# Autodesk Inventor part: PQ60 EPS FV4.brd_Outline
Saved by Autodesk Inventor 2015 SP1 (Build 190203100, 203)
## iProperties
Created: 2015-10-19
Part Number: PQ60 EPS FV4.brd_Outline
Material: Generic
Document SubType Name: Modeling
Designer: Kartikye
Density: 1 g/cm^3
Appearance: Board Outline
Author: Kartikye
Autodesk Inventor part; units mm, degrees
ref_plane "YZ Plane" through (0, 0, 0) normal (1, 0, 0) x (0, 1, 0)
ref_plane "XZ Plane" through (0, 0, 0) normal (0, 1, 0) x (-1, 0, 0)
ref_plane "XY Plane" through (0, 0, 0) normal (0, 0, 1) x (1, 0, 0)
sketch "Sketch1" plane through (0, 0, 0) normal (0, 0, 1) x (1, 0, 0)
  line L0 (42, 3) -> (42, 39)
  line L1 (42, 39) -> (41.8978, 39.7765)
  line L2 (41.8978, 39.7765) -> (41.5981, 40.5)
  line L3 (41.5981, 40.5) -> (41.1213, 41.1213)
  line L4 (41.1213, 41.1213) -> (40.5, 41.5981)
  line L5 (40.5, 41.5981) -> (39.7765, 41.8978)
  line L6 (39.7765, 41.8978) -> (39, 42)
  line L7 (39, 42) -> (3, 42)
  line L8 (3, 42) -> (2.2235, 41.8978)
  line L9 (2.2235, 41.8978) -> (1.5, 41.5981)
  line L10 (1.5, 41.5981) -> (0.8787, 41.1213)
  line L11 (0.8787, 41.1213) -> (0.4019, 40.5)
  line L12 (0.4019, 40.5) -> (0.1022, 39.7765)
  line L13 (0.1022, 39.7765) -> (0, 39)
  line L14 (0, 39) -> (0, 3)
  line L15 (0, 3) -> (0.1022, 2.2235)
  line L16 (0.1022, 2.2235) -> (0.4019, 1.5)
  line L17 (0.4019, 1.5) -> (0.8787, 0.8787)
  line L18 (0.8787, 0.8787) -> (1.5, 0.4019)
  line L19 (1.5, 0.4019) -> (2.2235, 0.1022)
  line L20 (2.2235, 0.1022) -> (3, 0)
  line L21 (3, 0) -> (39, 0)
  line L22 (39, 0) -> (39.7765, 0.1022)
  line L23 (39.7765, 0.1022) -> (40.5, 0.4019)
  line L24 (40.5, 0.4019) -> (41.1213, 0.8787)
  line L25 (41.1213, 0.8787) -> (41.5981, 1.5)
  line L26 (41.5981, 1.5) -> (41.8978, 2.2235)
  line L27 (41.8978, 2.2235) -> (42, 3)
  circle A0 centre (32.1, 8.8) radius 0.55
  circle A1 centre (9.9, 8.8) radius 0.35
  circle A2 centre (32.1, 8.5) radius 0.55
  circle A3 centre (9.9, 8.5) radius 0.35
  circle A4 centre (14.1, 12.1) radius 0.15
  circle A5 centre (16, 13.35) radius 0.15
  circle A6 centre (29.7, 2.6) radius 0.15
  circle A7 centre (35.3, 30.85) radius 0.15
  circle A8 centre (11.6, 12.1) radius 0.15
  circle A9 centre (11.6, 13.7) radius 0.15
  circle A10 centre (40.65, 7.95) radius 0.15
  circle A11 centre (14.85, 15.6) radius 0.15
  circle A12 centre (12.025, 26.75) radius 0.15
  circle A13 centre (12.025, 32.45) radius 0.15
  circle A14 centre (23.75, 32.425) radius 0.15
  circle A15 centre (30.6, 9.2) radius 0.15
  circle A16 centre (27.75, 11.25) radius 0.15
  circle A17 centre (24.9, 11.3) radius 0.15
  circle A18 centre (37.05, 26.85) radius 0.15
  circle A19 centre (24.9, 1.8) radius 0.15
  circle A20 centre (13.5, 12.9) radius 0.15
  circle A21 centre (17.1, 11.975) radius 0.15
  circle A22 centre (20.2, 11.975) radius 0.15
  circle A23 centre (23.3, 11.975) radius 0.15
  circle A24 centre (10.9, 12.9) radius 0.15
  circle A25 centre (22.5, 11.25) radius 0.15
  circle A26 centre (19.5, 11.3) radius 0.15
  circle A27 centre (17.7, 11.25) radius 0.15
  circle A28 centre (19.15, 25.175) radius 0.15
  circle A29 centre (3, 39) radius 1
  circle A30 centre (3, 3) radius 1
  circle A31 centre (39, 3) radius 1
  circle A32 centre (31.1, 7.05) radius 0.15
  circle A33 centre (7, 7.05) radius 0.15
  circle A34 centre (5.6, 7.05) radius 0.15
  circle A35 centre (13.5, 11.3) radius 0.15
  circle A36 centre (10.375, 36.875) radius 0.15
  circle A37 centre (20.85, 36.95) radius 0.15
  circle A38 centre (24.9, 36.275) radius 0.15
  circle A39 centre (30.55, 36.7) radius 0.15
  circle A40 centre (6, 18.6) radius 0.15
  circle A41 centre (30.95, 24.55) radius 0.15
  circle A42 centre (34.8, 23.4) radius 0.15
  circle A43 centre (10.9, 23.3) radius 0.15
  circle A44 centre (8.75, 23.4) radius 0.15
  circle A45 centre (14.2, 24.6) radius 0.15
  circle A46 centre (14.1, 22.25) radius 0.15
  circle A47 centre (18, 13.35) radius 0.15
  circle A48 centre (21.1, 13.35) radius 0.15
  circle A49 centre (16, 16.15) radius 0.15
  circle A50 centre (13.9, 14.3) radius 0.15
  circle A51 centre (19.375, 15.975) radius 0.15
  circle A52 centre (24.25, 13.4) radius 0.15
  circle A53 centre (27.35, 13.35) radius 0.15
  circle A54 centre (30.35, 12.1) radius 0.15
  circle A55 centre (34.9, 14.1) radius 0.15
  circle A56 centre (35.25, 7.7) radius 0.15
  circle A57 centre (40.675, 13.725) radius 0.15
  circle A58 centre (34.475, 21.275) radius 0.15
  circle A59 centre (38.225, 13.95) radius 0.15
  circle A60 centre (22.325, 27.6) radius 0.15
  circle A61 centre (9.8, 26.075) radius 0.15
  circle A62 centre (13.175, 27.15) radius 0.15
  circle A63 centre (27, 19.525) radius 0.15
  circle A64 centre (23.875, 15.75) radius 0.15
  circle A65 centre (29.525, 21.15) radius 0.15
  circle A66 centre (29.475, 27.45) radius 0.15
  circle A67 centre (31.675, 0.775) radius 0.15
  circle A68 centre (2.45, 8.075) radius 0.15
  circle A69 centre (39, 26.85) radius 0.15
  circle A70 centre (11.975, 35.375) radius 0.15
  circle A71 centre (6.2, 36.55) radius 0.15
  circle A72 centre (25.2, 32.45) radius 0.15
  circle A73 centre (34.5, 36.7) radius 0.15
  circle A74 centre (13.1, 30.875) radius 0.15
  circle A75 centre (6.6, 14.5) radius 0.15
  circle A76 centre (20.7, 2.7) radius 0.15
  circle A77 centre (9.05, 27.55) radius 0.15
  circle A78 centre (14.1, 19) radius 0.15
  circle A79 centre (15.3, 12.025) radius 0.15
  circle A80 centre (14.7, 11.3) radius 0.15
  circle A81 centre (14.1, 1.9) radius 0.15
  circle A82 centre (14.7, 2.7) radius 0.15
  circle A83 centre (15.3, 1.9) radius 0.15
  circle A84 centre (15.9, 2.7) radius 0.15
  circle A85 centre (16.5, 1.9) radius 0.15
  circle A86 centre (17.1, 2.7) radius 0.15
  circle A87 centre (17.7, 1.9) radius 0.15
  circle A88 centre (18.3, 2.7) radius 0.15
  circle A89 centre (18.9, 1.9) radius 0.15
  circle A90 centre (19.5, 2.7) radius 0.15
  circle A91 centre (20.1, 1.9) radius 0.15
  circle A92 centre (12.9, 1.9) radius 0.15
  circle A93 centre (12.2977, 2.7) radius 0.15
  circle A94 centre (19.8, 35.7) radius 0.15
  circle A95 centre (31.525, 35.675) radius 0.15
  circle A96 centre (9.05, 35.6) radius 0.15
  circle A97 centre (33.45, 24.65) radius 0.15
  circle A98 centre (3.15, 34.1) radius 0.15
  circle A99 centre (3.15, 27.45) radius 0.15
  circle A100 centre (14.9, 27.45) radius 0.15
  circle A101 centre (14.9, 34.1) radius 0.15
  circle A102 centre (3.7, 26.1) radius 0.15
  circle A103 centre (26.6, 34.1) radius 0.15
  circle A104 centre (26.6, 27.45) radius 0.15
  circle A105 centre (8.3, 20.75) radius 0.15
  circle A106 centre (37.075, 28.875) radius 0.15
  circle A107 centre (3.125, 20.5) radius 0.15
  circle A108 centre (1.725, 22.675) radius 0.15
  circle A109 centre (4.5, 16.8) radius 0.15
  circle A110 centre (6.4, 25.925) radius 0.15
  circle A111 centre (33.5, 23.45) radius 0.15
  circle A112 centre (37.125, 22.45) radius 0.15
  circle A113 centre (38.65, 16.075) radius 0.15
  circle A114 centre (33.65, 17.45) radius 0.15
  circle A115 centre (36.2, 15.75) radius 0.15
  circle A116 centre (22.6, 15.225) radius 0.15
  circle A117 centre (20.725, 17.575) radius 0.15
  circle A118 centre (25.75, 15.225) radius 0.15
  circle A119 centre (6.4, 25.05) radius 0.15
  circle A120 centre (10.875, 24.95) radius 0.15
  circle A121 centre (25.65, 0.6) radius 0.15
  circle A122 centre (5.7, 11.45) radius 0.15
  circle A123 centre (5.7, 12.45) radius 0.15
  circle A124 centre (10.5, 16.8) radius 0.15
  circle A125 centre (24.975, 17.5) radius 0.15
  circle A126 centre (18.125, 15.225) radius 0.15
  circle A127 centre (15.45, 17.5) radius 0.15
  circle A128 centre (37.3, 7.25) radius 0.15
  circle A129 centre (37.15, 9) radius 0.15
  circle A130 centre (28.9, 15.225) radius 0.15
  circle A131 centre (29.2, 17.45) radius 0.15
  circle A132 centre (12.7, 36.425) radius 0.15
  circle A133 centre (7.5, 37.275) radius 0.15
  circle A134 centre (33.55, 10.15) radius 0.15
  circle A135 centre (32.85, 12.05) radius 0.15
  circle A136 centre (23.1, 36.45) radius 0.15
  circle A137 centre (17.9, 37.275) radius 0.15
  circle A138 centre (33.5, 36.4) radius 0.15
  circle A139 centre (28.3, 37.3) radius 0.15
  circle A140 centre (39, 39) radius 1
  circle A141 centre (4.3, 36.1) radius 0.15
  circle A142 centre (13.3, 39.85) radius 0.15
  circle A143 centre (7.975, 40.075) radius 0.15
  circle A144 centre (16.075, 36.675) radius 0.15
  circle A145 centre (23.7, 39.85) radius 0.15
  circle A146 centre (18.25, 40.075) radius 0.15
  circle A147 centre (34.225, 39.825) radius 0.15
  circle A148 centre (29.475, 40.75) radius 0.15
  circle A149 centre (27.6, 35.65) radius 0.15
  circle A150 centre (13.5, 2.7) radius 0.15
  circle A151 centre (12.9, 12.1) radius 0.15
  circle A152 centre (13.5625, 19.9) radius 0.15
  circle A153 centre (12.3, 11.3) radius 0.15
  circle A154 centre (13.5625, 20.75) radius 0.15
  circle A155 centre (27.9, 21.75) radius 0.15
  circle A156 centre (32.5, 16.05) radius 0.15
  circle A157 centre (32.85, 22.15) radius 0.15
  circle A158 centre (25.9, 12.05) radius 0.15
  circle A159 centre (29.75, 14.375) radius 0.15
  circle A160 centre (30.95, 21.15) radius 0.15
  circle A161 centre (35.7, 17.5) radius 0.15
  constraints: 162 centre point, 56 end point
extrude "PQ60 EPS FV4.brd_Outline" add sketch "Sketch1" along normal blind 1
body "Solid1"
